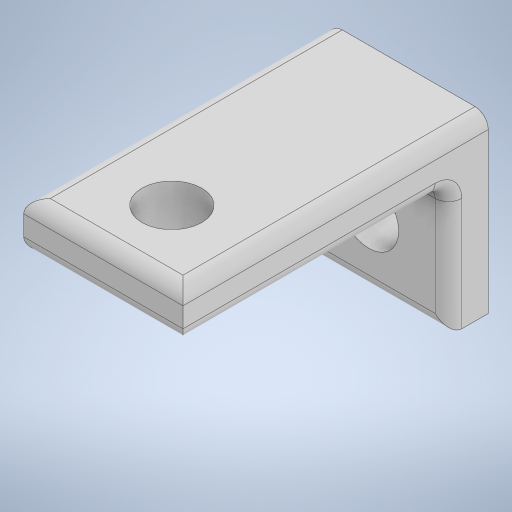
# Autodesk Inventor part: psu-bracket
Saved by Autodesk Inventor 2024 (Build 280153000, 153)
## iProperties
Created: 2024-05-11
Part Number: psu-bracket
Material: Generic
Document SubType Name: Modeling
Designer: MaartenGeorgesBuelen
Density: 1 g/cm^3
Appearance: Default
Author: MaartenGeorgesBuelen
## iProperties of the stored document psu-bracket_3DPrint.ipt
Created: 2024-05-11
Part Number: psu-bracket_3DPrint
Material: Generic
Document SubType Name: Modeling
Designer: MaartenGeorgesBuelen
Density: 1 g/cm^3
Appearance: Default
Author: MaartenGeorgesBuelen
Autodesk Inventor part; units mm, degrees
ref_plane "YZ Plane" through (0, 0, 0) normal (1, 0, 0) x (0, 1, 0)
ref_plane "XZ Plane" through (0, 0, 0) normal (0, 1, 0) x (-1, 0, 0)
ref_plane "XY Plane" through (0, 0, 0) normal (0, 0, 1) x (1, 0, 0)
sketch "Sketch1" plane through (0, 0, 0) normal (0, 0, 1) x (1, 0, 0)
  circle A0 centre (0, 0) radius 2.25
  line L0 (-6, 4.5) -> (6, 4.5)
  line L1 (6, 4.5) -> (6, -5)
  line L2 (6, -5) -> (-6, -5)
  line L3 (-6, -5) -> (-6, 4.5)
  line L4 (-6, 4.5) -> (6, 4.5)
  line L5 (6, 4.5) -> (6, 8)
  line L6 (6, 8) -> (-6, 8)
  line L7 (-6, 8) -> (-6, 4.5)
  dimension "d0" = 4.5
  dimension "d1" = 5
  dimension "d2" = 6
  dimension "d3" = 6
  dimension "d4" = 4.5
  dimension "d5" = 3.5
  constraints: 16 end point, 4 parallel, 2 horizontal, 2 perpendicular, 1 centre point, 1 coincident
  measures "d0" diameter of A0
  measures "d1" distance from line of L2 point (0, 0)
  measures "d2" distance from line of L3 point (0, 0)
  measures "d3" distance from line of L1 point (0, 0)
  measures "d4" distance from line of L0 point (0, 0)
  measures "d5" distance of L5.end L4.end
extrude "Extrusion1" add sketch "Sketch1" along normal blind 3
sketch "Sketch2" plane through (0, 0, 3) normal (0, 0, 1) x (1, 0, 0)
  line L0 (-6, -5) -> (6, -5) projected
  line L1 (6, -5) -> (6, 8) projected
  line L2 (6, 8) -> (-6, 8) projected
  line L3 (-6, 8) -> (-6, -5) projected
  circle A0 centre (0, 0) radius 2.25 projected
  line L4 (6, 8) -> (-6, 8) projected
  line L5 (-6, 8) -> (6, 8)
  line L6 (6, 8) -> (6, 4.5)
  line L7 (6, 4.5) -> (-6, 4.5)
  line L8 (-6, 4.5) -> (-6, 8)
  dimension "d8" = 3.5
  constraints: 8 end point, 2 parallel, 1 horizontal, 1 perpendicular, 1 point on line
  measures "d8" distance of L5.end L6.end
extrude "Extrusion2" add sketch "Sketch2" along normal blind 20 contours L3 L2 L1 L7
sketch "Sketch3" plane through (-6, 8, 0) normal (0, 1, 0) x (1, 0, 0)
  point P0 (6, 0)
  point P1 (6.0288, -17.8643)
hole "Hole1" at (0.0288, 8, 17.8643) direction (0, -1, 0) diameter 4.5 depth 4 tip angle 118
fillet "Fillet1" radius 1 10 edges at (0, 4.5, 3) (0, 8, 23) (0, 4.5, 23) (0, -5, 3) (-6, -0.25, 3) (6, -0.25, 3) (6, 4.5, 13) (-6, 4.5, 13) (-6, 8, 11.5) (6, 8, 11.5)
body "Solid1"
